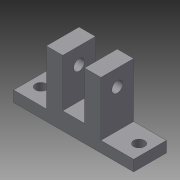
# Autodesk Inventor part: Arm_Pulley_Connector
Saved by Autodesk Inventor 2015 (Build 190159000, 159)
## iProperties
Created: 2017-03-09
Part Number: Arm_Pulley_Connector
Material: Generic
Document SubType Name: Modeling
Designer: Guy
Density: 1 g/cm^3
Appearance: Default
Author: Guy
Autodesk Inventor part; units mm, degrees
ref_plane "YZ Plane" through (0, 0, 0) normal (1, 0, 0) x (0, 1, 0)
ref_plane "XZ Plane" through (0, 0, 0) normal (0, 1, 0) x (-1, 0, 0)
ref_plane "XY Plane" through (0, 0, 0) normal (0, 0, 1) x (1, 0, 0)
sketch "Sketch1" plane through (0, 0, 0) normal (0, 0, 1) x (1, 0, 0)
  line L0 (0, 0) -> (25, 0)
  line L1 (25, 0) -> (25, 15)
  line L2 (25, 15) -> (0, 15)
  line L3 (0, 15) -> (0, 0)
  dimension "d0" = 25
  dimension "d1" = 15
  constraints: 8 end point, 2 parallel, 1 horizontal, 1 perpendicular
  measures "d0" distance of L2.end L1.end
  measures "d1" distance of L2.end L0.start
extrude "Extrusion1" add sketch "Sketch1" along normal blind 30
sketch "Sketch2" plane through (0, 15, 0) normal (0, 1, 0) x (1, 0, 0)
  line L0 (25, 0) -> (0, 0) projected
  line L1 (0, 0) -> (0, -30) projected
  line L2 (25, -30) -> (0, -30) projected
  line L3 (25, 0) -> (25, -30) projected
  line L4 (7.5, -30) -> (17.5, -30)
  line L5 (17.5, -30) -> (17.5, -8)
  line L6 (17.5, -8) -> (7.5, -8)
  line L7 (7.5, -8) -> (7.5, -30)
  point P0 (0, 0)
  dimension "d5" = 10
  dimension "d6" = 7.5
  dimension "d7" = 22
  constraints: 8 end point, 2 parallel, 1 horizontal, 1 perpendicular, 1 point on line
  measures "d5" distance between parallel lines of L5 L7
  measures "d6" distance between parallel lines of L7 L1
  measures "d7" distance between parallel lines of L2 L6
extrude "Extrusion2" cut sketch "Sketch2" against normal up to next contours L2 L7 L6 L5
sketch "Sketch3" plane through (25, 0, 0) normal (1, 0, 0) x (0, 0, -1)
  circle A0 centre (-22.5, 7.5) radius 2.5
  line L0 (-30, 0) -> (-30, 15) projected
  line L1 (0, 15) -> (-30, 15) projected
  point P0 (0, 0)
  dimension "d10" = 5
  dimension "d11" = 7.5
  dimension "d12" = 7.5
  constraints: 1 centre point
  measures "d10" diameter of A0
  measures "d11" distance from line of L0 A0.centre
  measures "d12" distance from line of L1 A0.centre
extrude "Extrusion3" cut sketch "Sketch3" against normal through all
sketch "Sketch4" plane through (0, 0, 0) normal (0, 0, -1) x (-1, 0, 0)
  line L0 (0, 0) -> (-25, 0) projected
  line L1 (0, 15) -> (0, 0) projected
  line L2 (-25, 15) -> (0, 15) projected
  line L3 (-25, 0) -> (-25, 15) projected
  line L4 (-25, 15) -> (-40, 15)
  line L5 (-40, 15) -> (-40, 0)
  line L6 (-40, 0) -> (-25, 0)
  line L7 (-25, 0) -> (-25, 15)
  line L8 (0, 15) -> (15, 15)
  line L9 (15, 15) -> (15, 0)
  line L10 (15, 0) -> (0, 0)
  line L11 (0, 0) -> (0, 15)
  dimension "d15" = 15
  dimension "d16" = 15
  constraints: 16 end point, 4 parallel, 2 horizontal, 2 perpendicular, 1 point on line
  measures "d15" distance of L1.start L8.end
  measures "d16" distance of L2.start L4.end
extrude "Extrusion4" add sketch "Sketch4" against normal blind 5 contours L1 L8 L9 L10 | L6 L5 L4 L3
sketch "Sketch5" plane through (0, 0, 5) normal (0, 0, 1) x (1, 0, 0)
  circle A0 centre (-10, 7.5) radius 2.5
  circle A1 centre (35, 7.5) radius 2.5
  line L0 (0, 15) -> (-15, 15) projected
  line L1 (40, 15) -> (25, 15) projected
  line L2 (40, 0) -> (40, 15) projected
  line L3 (-15, 15) -> (-15, 0) projected
  point P0 (0, 0)
  dimension "d19" = 5
  dimension "d20" = 5
  dimension "d21" = 7.5
  dimension "d22" = 7.5
  dimension "d23" = 5
  dimension "d24" = 5
  constraints: 2 centre point
  measures "d19" diameter of A1
  measures "d20" diameter of A0
  measures "d21" distance from line of A0.centre L0
  measures "d22" distance from line of A1.centre L1
  measures "d23" distance from line of A1.centre L2
  measures "d24" distance from line of A0.centre L3
extrude "Extrusion5" cut sketch "Sketch5" against normal up to next
body "Solid1"
